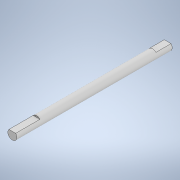
# Autodesk Inventor part: Ось 3мм задняя
Saved by Autodesk Inventor 2020 (Build 240168000, 168)
## iProperties
Created: 2021-03-15
Part Number: Ось 3мм задняя
Material: Типовые
Document SubType Name: ЛистМат
Designer: Антон
Density: 1 g/cm^3
Appearance: По умолчанию
Mass: 0.401662 g
Surface Area: 5.5565 cm^2
Volume: 0.401662 cm^3
Sheet Metal Rule: По умолчанию
Author: Антон
Autodesk Inventor part; units mm, degrees
ref_plane "YZ Plane" through (0, 0, 0) normal (1, 0, 0) x (0, 1, 0)
ref_plane "XZ Plane" through (0, 0, 0) normal (0, 1, 0) x (-1, 0, 0)
ref_plane "XY Plane" through (0, 0, 0) normal (0, 0, 1) x (1, 0, 0)
sketch "Эскиз1" plane through (0, 0, 0) normal (0, 0, 1) x (1, 0, 0)
  circle A0 centre (0, 0) radius 1.5
  dimension "d0" = 3
  constraints: 1 centre point, 1 coincident
  measures "d0" diameter of A0
extrude "Выдавливание1" add sketch "Эскиз1" along normal blind 51.25
sketch "Эскиз2" plane through (0, 0, 51.25) normal (0, 0, 1) x (1, 0, 0)
  line L0 (-1.5, -1) -> (1.5, -1)
  line L1 (1.5, -1) -> (1.5, 1)
  line L2 (1.5, 1) -> (-1.5, 1)
  line L3 (-1.5, 1) -> (-1.5, -1)
  line L4 (-1.5, -1) -> (1.5, 1) construction
  line L5 (1.5, -1) -> (-1.5, 1) construction
  circle A0 centre (0, 0) radius 1.5
  point P0 (-1.118, 1)
  point P1 (1.118, 1)
  dimension "d3" = 2
  constraints: 12 end point, 2 midpoint, 2 parallel, 1 centre point, 1 coincident, 1 horizontal, 1 perpendicular
  measures "d3" distance of L1.end L0.end
extrude "Выдавливание2" cut sketch "Эскиз2" against normal blind 8 contours A0 L2
sketch "Эскиз3" plane through (0, 0, 0) normal (0, 0, -1) x (-1, 0, 0)
  arc A0 (1.118, 1) -> (-1.118, 1) centre (0, 0) ccw projected
  line L0 (-1.118, 1) -> (1.118, 1) projected
extrude "Выдавливание3" cut sketch "Эскиз3" against normal blind 5
equation "\"Радиус_гибки\" = Толщина"
equation "\"Ширина_просечки\" = Толщина"
equation "\"Глубина_просечки\" = 0.5 * Толщина"
equation "\"Размер_просечки\" = 4 * Толщина"
equation "\"Мин_остаток\" = 2 * Толщина"
equation "\"Радиус_перехода\" = Радиус_гибки"
equation "\"Радиус_Якоби\" = Толщина"
equation "\"Размер_зазора\" = Толщина"
equation "\"Толщина\" = 0.5"
